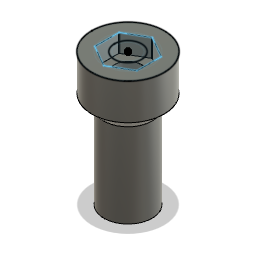
slim legs v2 (Autodesk Fusion 360 design; units mm, degrees)
Autodesk Fusion 360 part; units mm, degrees
sketch "Sketch1" plane through (0, 0, 0) normal (0, 1, 0) x (1, 0, 0)
  circle A0 centre (0, 0) radius 1.9
  circle A1 centre (0, 0) radius 4
  dimension "d1" = 3.8
  dimension "d2" = 8
  constraint coincident A0.centre A1.centre
  measures "d1" diameter of A0
  measures "d2" diameter of A1
extrude "Extrude1" add sketch "Sketch1" along normal blind 22
chamfer "Chamfer2" distance 0.5 angle 45 1 edges at (-1.7714, 0, -0.6871)
sketch "Sketch2" plane through (0, 22, 0) normal (0, 1, 0) x (-1, 0, 0)
  circle A0 centre (0, 0) radius 1.9
  circle A1 centre (0, 0) radius 4
  circle A2 centre (0, 0) radius 6
  line L0 (3.5, 2.0207) -> (0, 4.0415)
  line L1 (0, 4.0415) -> (-3.5, 2.0207)
  line L2 (-3.5, 2.0207) -> (-3.5, -2.0207)
  line L3 (-3.5, -2.0207) -> (0, -4.0415)
  line L4 (0, -4.0415) -> (3.5, -2.0207)
  line L5 (3.5, -2.0207) -> (3.5, 2.0207)
  circle A3 centre (0, 0) radius 2.25
  dimension "d7" = 12
  dimension "d8" = 3.5
  dimension "d9" = 4.5
  constraint concentric A0 A2
  constraint coincident A0.centre A1.centre
  measures "d7" diameter of A2
  measures "d8" distance of A0.centre L5
  measures "d9" diameter of A3
extrude "Extrude3" cut sketch "Sketch2" against normal blind 3 contours A1 L0 L1 L2 L3 L4 L5 | A3
extrude "Extrude2" add sketch "Sketch2" against normal blind 8 contours A1 L0 L5 | A1 L4 L5 | A1 L0 L1 | A1 L3 L4 | A1 L1 L2 | A1 L2 L3 | A2
extrude "Extrude4" cut sketch "Sketch2" against normal blind 10 contours A3
chamfer "Chamfer3" distance 2 angle 45 1 edges at (5.594, 14, 2.1697)
chamfer "Chamfer4" distance 0.3 angle 45 1 edges at (-1.7714, 12, 0.6871)
